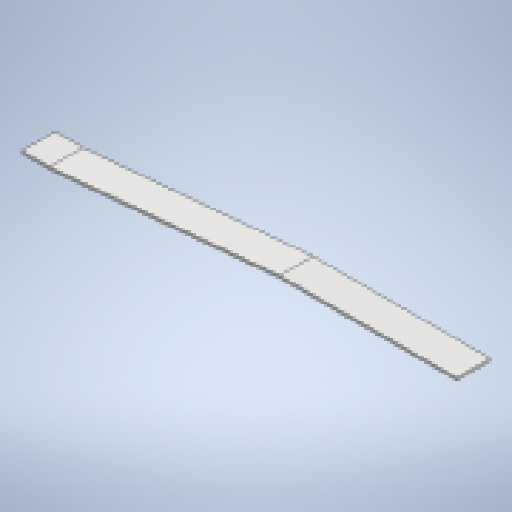
# Autodesk Inventor part: bok2
Saved by Autodesk Inventor 2023 (Build 270158000, 158)
## iProperties
Created: 2023-05-31
Part Number: bok2
Material: Ogólny
Document SubType Name: Modeling
Designer: Kamil
Density: 1 g/cm^3
Appearance: Domyślna
Author: Kamil
Autodesk Inventor part; units mm, degrees
ref_plane "YZ Plane" through (0, 0, 0) normal (1, 0, 0) x (0, 1, 0)
ref_plane "XZ Plane" through (0, 0, 0) normal (0, 1, 0) x (-1, 0, 0)
ref_plane "XY Plane" through (0, 0, 0) normal (0, 0, 1) x (1, 0, 0)
sketch "Szkic1" plane through (0, 0, 0) normal (0, 0, 1) x (1, 0, 0)
  line L0 (46.9852, 26.6235) -> (8.5048, 23.1186) projected
  line L1 (-61.9852, 19.3198) -> (-38.201, 19.3198) projected
  line L2 (-33.201, 19.3198) -> (-38.201, 19.3198) projected
  line L3 (-61.9852, 19.3198) -> (-66.9852, 19.3198) projected
  line L4 (46.9852, 26.6235) -> (-33.201, 19.3198)
  line L5 (46.9852, 26.6235) -> (243.11, 44.4876)
  line L6 (8.5048, 1) -> (16.799, 1) projected
  line L7 (8.5048, -1) -> (16.799, -1) projected
  line L8 (243.1277, 44.4876) -> (455.4993, 44.4876)
  line L9 (-66.9852, 19.3198) -> (-33.201, 19.3198)
  line L10 (243.2412, 47.4876) -> (455.4993, 47.4876)
  line L11 (242.9736, 47.4876) -> (46.713, 29.6112)
  line L12 (46.713, 29.6112) -> (-33.4732, 22.3074)
  line L13 (-33.4732, 22.3074) -> (-66.9852, 22.3074)
  line L14 (-66.9852, 22.3074) -> (-66.9852, 19.3198)
  line L15 (455.4993, 47.4876) -> (455.4993, 44.4876)
  line L16 (243.2412, 47.4876) -> (242.9736, 47.4876)
  line L17 (243.1277, 44.4876) -> (243.11, 44.4876)
  point P0 (0, 0)
  dimension "d1" = 3
  dimension "d2" = 3
  constraints: 24 end point, 4 horizontal, 2 collinear, 2 point on line, 1 parallel, 1 perpendicular, 1 vertical, 1 other
  measures "d1" distance between parallel lines of L8 L10
  measures "d2" distance between parallel lines of L5 L11
extrude "Wyciągnięcie proste1" add sketch "Szkic1" against normal blind 40
fillet "Zaokrąglenie1" radius 20 2 edges at (-66.9852, 20.8136, 0) (-66.9852, 20.8136, -40)
